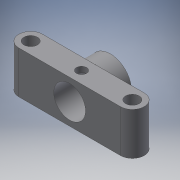
# Autodesk Inventor part: reed switch holder
Saved by Autodesk Inventor 2016 (Build 200138000, 138)
## iProperties
Created: 2017-08-17
Part Number: reed switch holder
Material: Generic
Document SubType Name: Modeling
Designer: zimirken
Density: 1 g/cm^3
Appearance: Default
Author: zimirken
Autodesk Inventor part; units mm, degrees
ref_plane "YZ Plane" through (0, 0, 0) normal (1, 0, 0) x (0, 1, 0)
ref_plane "XZ Plane" through (0, 0, 0) normal (0, 1, 0) x (-1, 0, 0)
ref_plane "XY Plane" through (0, 0, 0) normal (0, 0, 1) x (1, 0, 0)
sketch "Sketch1" plane through (0, 0, 0) normal (0, 0, 1) x (1, 0, 0)
  line L0 (-30, 0) -> (30, 0) construction
  circle A0 centre (-30, 0) radius 4
  circle A1 centre (30, 0) radius 4
  line L1 (-30, 0) -> (30, 0) construction
  line L2 (-30, -7) -> (30, -7)
  line L3 (30, 7) -> (-30, 7)
  arc A2 (-30, 7) -> (-30, -7) centre (-30, 0) ccw
  arc A3 (30, -7) -> (30, 7) centre (30, 0) ccw
  point P0 (0, 0)
  point P1 (0, 0)
  point P2 (0, 0)
  dimension "d0" = 60
  dimension "d1" = 8
  dimension "d2" = 7
  constraints: 10 end point, 4 centre point, 4 point on circle, 4 tangent, 3 coincident, 2 equal length, 2 midpoint, 1 equal radius, 1 horizontal
  measures "d0" distance of L0.start L0.end
  measures "d1" diameter of A0
  measures "d2" radius of A2
extrude "Extrusion1" add sketch "Sketch1" along normal blind 25
sketch "Sketch2" plane through (-30, -7, 0) normal (0, -1, 0) x (1, 0, 0)
  line L0 (0, 0) -> (60, 0) construction
  line L1 (60, 0) -> (60, 25) construction
  line L2 (0, 25) -> (60, 25) construction
  line L3 (0, 0) -> (0, 25) construction
  line L4 (30, 25) -> (30, 0) construction
  circle A0 centre (30, 12.5) radius 9.375
  dimension "d5" = 18.75
  constraints: 2 end point, 2 midpoint, 1 centre point, 1 vertical
  measures "d5" diameter of A0
extrude "Extrusion2" cut sketch "Sketch2" against normal through all
sketch "Sketch3" plane through (-30, 7, 0) normal (0, 1, 0) x (1, 0, 0)
  circle A0 centre (30, -12.5) radius 9.375 projected
  circle A1 centre (30, -12.5) radius 12.5
  line L0 (60, -25) -> (0, -25) projected
  point P0 (30, 0)
  constraints: 1 centre point, 1 coincident, 1 tangent
extrude "Extrusion3" add sketch "Sketch3" along normal blind 10
sketch "Sketch4" plane through (0, 0, 25) normal (0, 0, 1) x (1, 0, 0)
  circle A0 centre (0, 0) radius 3
  dimension "d10" = 6
  constraints: 1 centre point, 1 coincident
  measures "d10" diameter of A0
extrude "Extrusion4" cut sketch "Sketch4" against normal up to next
body "Solid1"
